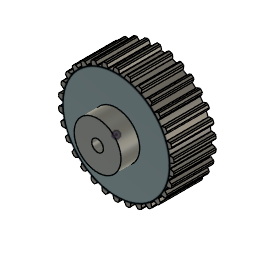
Gear_30 (Autodesk Fusion 360 design; units mm, degrees)
part number: 2026-07-17-20-20-12-851
Autodesk Fusion 360 part; units mm, degrees
sketch "Sketch1" plane through (0, 0, 0) normal (0, 1, 0) x (1, 0, 0)
  circle A0 centre (0, 0) radius 22.8
  dimension "d1" = 45.6
  constraint coincident A0.centre origin
  measures "d1" diameter of A0
extrude "Extrude1" add sketch "Sketch1" along normal blind 18 makes body 1
sketch "Sketch2" plane through (0, 0, 0) normal (0, -1, 0) x (1, 0, 0)
  circle A0 centre (0, 0) radius 22.8
  circle A1 centre (0, 0) radius 2.5
  dimension "d4" = 5
  constraint concentric A0 A1
  measures "d4" diameter of A1
extrude "Extrude2" cut sketch "Sketch2" against normal blind 65 contours A1 bodies 1
sketch "Sketch3" plane through (0, 0, 0) normal (0, -1, 0) x (1, 0, 0)
  circle A0 centre (0, 0) radius 2.5
  circle A1 centre (0, 0) radius 22.8
  circle A2 centre (0, 0) radius 10
  dimension "d7" = 20
  constraint coincident A0.centre A1.centre
  measures "d7" diameter of A2
extrude "Extrude3" add sketch "Sketch3" along normal blind 8 contours A2 bodies 1
sketch "Sketch5" plane through (0, 18, 0) normal (0, 1, 0) x (-1, 0, 0)
  circle A0 centre (0, 0) radius 2.5
  circle A1 centre (0, 0) radius 22.8
  circle A2 centre (0, 0) radius 22.8
  line L0 (-1.3883, 23.1344) -> (-1.0229, 24.3903)
  line L1 (-1.1003, 22.7506) -> (1.0933, 22.7506)
  line L2 (-0.5435, 24.7506) -> (0.5131, 24.7506)
  line L3 (0.9908, 24.3982) -> (1.3799, 23.1392)
  arc A3 (-0.5435, 24.7506) -> (-1.0229, 24.3903) centre (-0.5428, 24.2506) ccw
  arc A4 (0.9908, 24.3982) -> (0.5131, 24.7506) centre (0.5131, 24.2506) ccw
  arc A5 (-1.3883, 23.1344) -> (-1.1003, 22.7506) centre (-1.1003, 23.0506) ccw
  arc A6 (1.0933, 22.7506) -> (1.3799, 23.1392) centre (1.0933, 23.0506) ccw
  point P0 (-1.5, 22.7506)
  point P1 (-0.918, 24.7506)
  point P2 (1.5, 22.7506)
  point P3 (0.882, 24.7506)
  dimension "d28" = 3
  dimension "d29" = 1.8
  dimension "d31" = 2
  dimension "d32" = 0.5
  dimension "d33" = 0.5
  dimension "d34" = 0.3
  constraint coincident A2 P0
  constraint horizontal L1
  constraint horizontal L2
  constraint coincident A2 P2
  constraint coincident P1 L0
  constraint coincident P1 L2
  constraint tangent L0 A3
  constraint coincident P3 L2
  constraint coincident P3 L3
  constraint tangent L2 A4
  constraint tangent L3 A4
  constraint coincident P0 L0
  constraint coincident P0 L1
  constraint tangent L0 A5
  constraint tangent L1 A5
  constraint coincident P2 L1
  constraint coincident P2 L3
  constraint tangent L1 A6
  constraint tangent L3 A6
  constraint equal A5 A6
  measures "d28" distance of P0 P2
  measures "d29" distance of P1 P3
  measures "d31" distance of L1 L2
  measures "d32" radius of A3
  measures "d33" radius of A4
  measures "d34" radius of A5
extrude "Extrude7" add sketch "Sketch5" against normal blind 18 separate body contours A1 A2 L0 L2 L3 A3 A4 A5 A6 makes body 2
pattern_circular "C-Pattern3" count 30 over 360 about axis through (0, 18, 0) along (0, -1, 0) of "Extrude7" makes body 3 makes body 4 makes body 5 makes body 6 makes body 7 makes body 8 makes body 9 makes body 10 makes body 11 makes body 12 makes body 13 makes body 14 makes body 15 makes body 16 makes body 17 makes body 18 makes body 19 makes body 20 makes body 21 makes body 22 makes body 23 makes body 24 makes body 25 makes body 26 makes body 27 makes body 28 makes body 29 makes body 30 makes body 31
